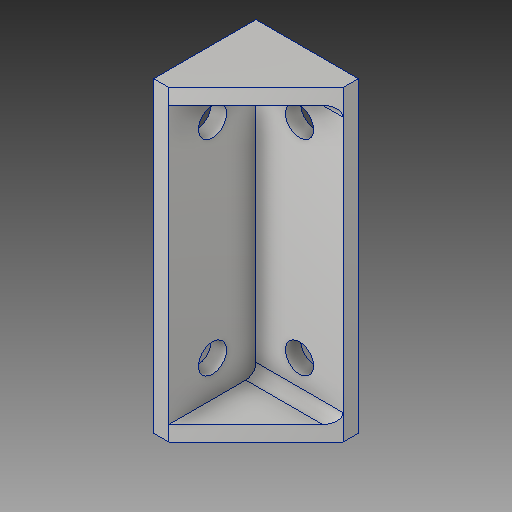
# Autodesk Inventor part: 2060 Custom Bracing
Saved by Autodesk Inventor 2019.4 (Build 234330000, 330)
## iProperties
Created: 2020-01-01
Part Number: 2060 Custom Bracing
Material: Aluminum 6061
Document SubType Name: Modeling
Designer: Mark
Mass: 19.6299 g
Surface Area: 55.2849 cm^2
Volume: 7.27032 cm^3
Density: 2.7 g/cm^3
Appearance: Aluminum - Flat
Author: Mark
Autodesk Inventor part; units mm, degrees
ref_plane "YZ Plane" through (0, 0, 0) normal (1, 0, 0) x (0, 1, 0)
ref_plane "XZ Plane" through (0, 0, 0) normal (0, 1, 0) x (-1, 0, 0)
ref_plane "XY Plane" through (0, 0, 0) normal (0, 0, 1) x (1, 0, 0)
sketch "Sketch1" plane through (0, 0, 0) normal (0, 0, 1) x (1, 0, 0)
  line L0 (-10, -30) -> (10, -30)
  line L1 (10, -30) -> (10, 30)
  line L2 (10, 30) -> (-10, 30)
  line L3 (-10, 30) -> (-10, -30)
  line L4 (-10, -30) -> (10, 30) construction
  line L5 (10, -30) -> (-10, 30) construction
  circle A0 centre (1.5, 20) radius 2.75
  circle A1 centre (1.5, -20) radius 2.75
  point P0 (0, 0)
  dimension "d0" = 20
  dimension "d1" = 60
  dimension "d20" = 5.5
  dimension "d21" = 5.5
  dimension "d22" = 10
  dimension "d23" = 8.5
  dimension "d24" = 8.5
  dimension "d25" = 10
  constraints: 12 end point, 2 centre point, 2 midpoint, 2 parallel, 1 horizontal, 1 perpendicular
  measures "d0" distance of L2.end L1.end
  measures "d1" distance of L1.end L0.end
  measures "d20" diameter of A0
  measures "d21" diameter of A1
  measures "d22" distance from line of L0 A1.centre
  measures "d23" distance from line of A1.centre L1
  measures "d24" distance from line of L1 A0.centre
  measures "d25" distance from line of L2 A0.centre
extrude "Extrusion1" add sketch "Sketch1" along normal blind 3
sketch "Sketch2" plane through (0, 0, 3) normal (0, 0, 1) x (1, 0, 0)
  line L0 (10, 30) -> (-10, 30) projected
  line L1 (-10, 30) -> (-7, 30)
  line L2 (-7, 30) -> (-7, -30)
  line L3 (-7, -30) -> (-10, -30)
  line L4 (-10, -30) -> (-10, 30)
  point P0 (0, 0)
  dimension "d4" = 3
  dimension "d5" = 60
  constraints: 8 end point, 2 parallel, 1 horizontal, 1 perpendicular
  measures "d4" distance of L2.end L3.end
  measures "d5" distance of L1.end L2.end
extrude "Extrusion2" add sketch "Sketch2" along normal blind 17
sketch "Sketch3" plane through (-10, 30, 0) normal (0, 1, 0) x (1, 0, 0)
  line L0 (0, 0) -> (20, 0)
  line L1 (20, 0) -> (20, -20)
  line L2 (20, -20) -> (0, -20)
  line L3 (0, -20) -> (0, 0)
  point P0 (10, 0)
  dimension "d8" = 20
  dimension "d9" = 20
  constraints: 8 end point, 2 parallel, 1 horizontal, 1 perpendicular
  measures "d8" distance of L1.end L2.end
  measures "d9" distance of L0.end L1.end
extrude "Extrusion3" add sketch "Sketch3" against normal blind 3
sketch "Sketch4" plane through (-10, -30, 0) normal (0, -1, 0) x (1, 0, 0)
  line L0 (0, 0) -> (20, 0)
  line L1 (20, 0) -> (20, 20)
  line L2 (20, 20) -> (0, 20)
  line L3 (0, 20) -> (0, 0)
  point P0 (10, 0)
  dimension "d12" = 20
  dimension "d13" = 20
  constraints: 8 end point, 2 parallel, 1 horizontal, 1 perpendicular
  measures "d12" distance of L2.end L1.end
  measures "d13" distance of L1.end L0.end
extrude "Extrusion4" add sketch "Sketch4" against normal blind 3
chamfer "Chamfer1" distance 17 angle 45 2 edges at (10, -28.5, 20) (10, 28.5, 20)
fillet "Fillet1" radius 2 2 edges at (1.5, 27, 3) (1.5, -27, 3)
sketch "Sketch5" plane through (-7, -27, 20) normal (1, 0, 0) x (0, 0, -1)
  circle A0 centre (8.5, 7) radius 2.75
  circle A1 centre (8.5, 47) radius 2.75
  line L0 (17, 57) -> (0, 57) projected
  line L1 (0, 0) -> (0, 54) projected
  line L2 (0, -3) -> (17, -3) projected
  point P0 (20, 27)
  dimension "d26" = 5.5
  dimension "d27" = 5.5
  dimension "d28" = 10
  dimension "d29" = 8.5
  dimension "d30" = 8.5
  dimension "d31" = 10
  constraints: 2 centre point
  measures "d26" diameter of A0
  measures "d27" diameter of A1
  measures "d28" distance from line of L0 A1.centre
  measures "d29" distance from line of L1 A1.centre
  measures "d30" distance from line of L1 A0.centre
  measures "d31" distance from line of L2 A0.centre
extrude "Extrusion5" cut sketch "Sketch5" against normal blind 3
body "Solid1"
